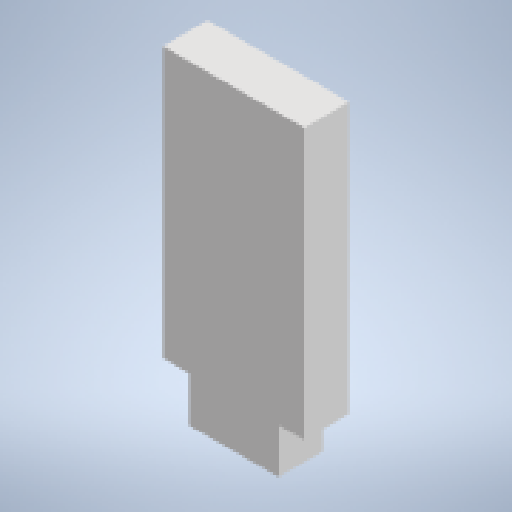
# Autodesk Inventor part: servo short side
Saved by Autodesk Inventor 2023 (Build 270158000, 158)
## iProperties
Created: 2023-10-15
Part Number: servo short side
Material: Generic
Document SubType Name: Modeling
Designer: Nate
Density: 1 g/cm^3
Appearance: Default
Author: Nate
Autodesk Inventor part; units mm, degrees
ref_plane "YZ Plane" through (0, 0, 0) normal (1, 0, 0) x (0, 1, 0)
ref_plane "XZ Plane" through (0, 0, 0) normal (0, 1, 0) x (-1, 0, 0)
ref_plane "XY Plane" through (0, 0, 0) normal (0, 0, 1) x (1, 0, 0)
sketch "Sketch1" plane through (0, 0, 0) normal (0, 0, 1) x (1, 0, 0)
  line L0 (0, 0) -> (12.7, 0)
  line L1 (12.7, 0) -> (12.7, 6.35)
  line L2 (12.7, 6.35) -> (0, 6.35)
  line L3 (0, 6.35) -> (0, 0)
  line L4 (-3.6576, 44.45) -> (16.3322, 44.45)
  line L5 (16.3322, 44.45) -> (16.3322, 6.35)
  line L6 (16.3322, 6.35) -> (-3.6576, 6.35)
  line L7 (-3.6576, 6.35) -> (-3.6576, 44.45)
  point P0 (16.3322, 25.4)
  point P1 (-3.6576, 25.4)
  dimension "d0" = 12.7
  dimension "d1" = 6.35
  dimension "d2" = 19.9898
  dimension "d3" = 3.6576
  dimension "d4" = 38.1
  constraints: 16 end point, 4 parallel, 2 horizontal, 2 midpoint, 2 perpendicular, 1 point on line
  measures "d0" distance of L2.end L1.end
  measures "d1" distance of L1.end L0.end
  measures "d2" distance of point (16.332, 25.4) point (-3.658, 25.4)
  measures "d3" distance between parallel lines of L7 L3
  measures "d4" distance between parallel lines of L4 L6
extrude "Extrusion1" add sketch "Sketch1" along normal blind 6.35
body "Solid1"
